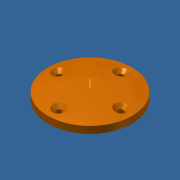
# Autodesk Inventor part: Abdeckung
Saved by Autodesk Inventor 2014 SP2 (Build 180246200, 246)
## iProperties
Created: 2014-12-12
Part Number: Abdeckung
Material: ABS-Kunststoff - Orange
Document SubType Name: Modeling
Designer: 4ndreas
Density: 1.06 g/cm^3
Appearance: Glatt - weiß(1)
Mass: 7.26906 g
Surface Area: 48.4344 cm^2
Volume: 6.8576 cm^3
Author: 4ndreas
Autodesk Inventor part; units mm, degrees
ref_plane "YZ Plane" through (0, 0, 0) normal (1, 0, 0) x (0, 1, 0)
ref_plane "XZ Plane" through (0, 0, 0) normal (0, 1, 0) x (-1, 0, 0)
sketch "Skizze1" plane through (0, 0, 0) normal (0, 0, 1) x (1, 0, 0)
  circle A0 centre (0, 18.125) radius 1.4 projected
  circle A1 centre (-18.125, 0) radius 1.4 projected
  circle A2 centre (0, -18.125) radius 1.4 projected
  circle A3 centre (18.125, 0) radius 1.4 projected
  circle A4 centre (0, 0) radius 11.25 projected
  circle A5 centre (0, 0) radius 25 projected
  circle A6 centre (0, 0) radius 24.5
  line L0 (-18.125, 0) -> (18.125, 0)
  circle A7 centre (0, 0) radius 13
  point P0 (0, 0)
  dimension "d0" = 49
  dimension "d19" = 26
  constraints: 2 centre point, 2 end point, 1 horizontal
  measures "d0" diameter of A6
  measures "d19" diameter of A7
extrude "Extrusion1" add sketch "Skizze1" along normal blind 4 contours A7 L0 A4 | L0 A4 A7 | A6
sketch "Skizze2" plane through (0, 0, 4) normal (0, 0, 1) x (1, 0, 0)
  circle A0 centre (0, 0) radius 11.25 projected
  circle A1 centre (18.125, 0) radius 1.4 projected
  circle A2 centre (0, -18.125) radius 1.4 projected
  circle A3 centre (-18.125, 0) radius 1.4 projected
  circle A4 centre (0, 18.125) radius 1.4 projected
  circle A5 centre (0, 0) radius 24.5 projected
ref_plane "Arbeitsebene1" through (-18.125, 0, 0) normal (0, -1, 0) x (1, 0, 0)
sketch "Skizze3" plane through (-18.125, 0, 0) normal (0, -1, 0) x (1, 0, 0)
  line L0 (34.85, 4) -> (34.85, 0) projected
  line L1 (34.85, 0) -> (29.375, 0) projected
  line L2 (29.375, 0) -> (29.375, 4) projected
  line L3 (29.375, 4) -> (34.85, 4) projected
  line L4 (1.4, 0) -> (1.4, 4) projected
  line L5 (1.4, 4) -> (6.875, 4) projected
  line L6 (6.875, 4) -> (6.875, 0) projected
  line L7 (6.875, 0) -> (1.4, 0) projected
  line L8 (-6.375, 0) -> (-6.375, 4) projected
  line L9 (-6.375, 4) -> (-1.4, 4) projected
  line L10 (-1.4, 4) -> (-1.4, 0) projected
  line L11 (-1.4, 0) -> (-6.375, 0) projected
  line L12 (42.625, 4) -> (42.625, 0) projected
  line L13 (42.625, 0) -> (37.65, 0) projected
  line L14 (37.65, 0) -> (37.65, 4) projected
  line L15 (37.65, 4) -> (42.625, 4) projected
  arc A0 (18.125, 6) -> (-6.375, 4) centre (18.125, -145.0625) ccw
  line L16 (18.125, 6) -> (18.125, 4)
  line L17 (18.125, 4) -> (-6.375, 4)
  line L18 (18.125, 18.126) -> (18.125, -80.6859)
  point P0 (18.125, 0)
  dimension "d4" = 2
  constraints: 6 end point, 2 collinear, 2 perpendicular, 2 point on circle, 2 point on line, 1 centre point, 1 vertical, 2 other
  measures "d4" distance from line of L17 L16.start
revolve "Umdrehung1" add sketch "Skizze3" angle 360 about axis through (0, 0, 6) along (0, 0, -1) contours L17 L9 A0 L16 L5
sketch "Skizze4" plane through (0, 0, 0) normal (0, 0, -1) x (-1, 0, 0)
  circle A0 centre (-18.125, 0) radius 1.4 projected
  circle A1 centre (0, -18.125) radius 1.4 projected
  circle A2 centre (18.125, 0) radius 1.4 projected
  circle A3 centre (0, 18.125) radius 1.4 projected
hole "Bohrung1" at (18.125, 0, 0) at (0, -18.125, 0) at (-18.125, 0, 0) at (0, 18.125, 0) direction (0, 0, 1) diameter 3.3 end through all
chamfer "Fase1" distance 2 angle 45 6 edges at (-16.961, 1.1694, 5.0403) (-19.2889, 1.1696, 4.7589) (-18.1249, -1.65, 4.8996) (0, 16.475, 5.0989) (18.1248, -1.65, 4.8997) (0, -19.775, 4.7001)
sketch "Skizze5" plane through (0, 0, 0) normal (0, 0, -1) x (-1, 0, 0)
  circle A0 centre (0, 0) radius 11.25 projected
  circle A1 centre (0, 0) radius 13.5
  dimension "d20" = 27
  constraints: 1 centre point
  measures "d20" diameter of A1
extrude "Extrusion2" cut sketch "Skizze5" against normal up to surface (4 mm away)
